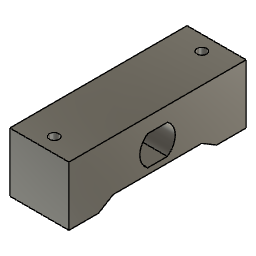
Motor mount test v1 (Autodesk Fusion 360 design; units mm, degrees)
Autodesk Fusion 360 part; units mm, degrees
sketch "Sketch1" plane through (0, 0, 0) normal (0, 0, 1) x (1, 0, 0)
  line L0 (0, 0) -> (20, 0)
  line L1 (20, 0) -> (20, 60)
  line L2 (20, 60) -> (0, 60)
  line L3 (0, 60) -> (0, 0)
  constraint horizontal L0
  constraint vertical L1
  constraint horizontal L2
  constraint vertical L3
  constraint coincident L0.start L3.end
extrude "Extrude1" add sketch "Sketch1" along normal blind 30
extrude "Extrude2" cut 1 faces at (6.6667, 40, 30) along direction (0, 0, -1) blind 10
sketch "Sketch2" plane through (20, 0, 0) normal (1, 0, 0) x (0, 1, 0)
  line L0 (60, 20) -> (0, 20)
  line L1 (0, 20) -> (0, 0)
  line L2 (0, 0) -> (60, 0)
  line L3 (60, 0) -> (60, 20)
  line L4 (36, 5) -> (24, 5)
  line L5 (24, 5) -> (24, 15)
  line L6 (24, 15) -> (36, 15)
  line L7 (36, 15) -> (36, 5)
  line L8 (36, 5) -> (24, 15) construction
  line L9 (24, 5) -> (36, 15) construction
  circle A0 centre (30, 10) radius 6
  point P0 (30, 10)
  constraint horizontal L4
  constraint perpendicular L4 L5
  constraint parallel L4 L6
  constraint parallel L5 L7
  constraint coincident L8 P0
  constraint coincident L9 P0
  constraint coincident P0 A0.centre
extrude "Extrude3" cut sketch "Sketch2" against normal blind 29 contours L4 L6 A0
sketch "Sketch3" plane through (0, 0, 0) normal (0, 0, -1) x (1, 0, 0)
  line L0 (0, 0) -> (0, -60)
  line L1 (0, -60) -> (20, -60)
  line L2 (20, -60) -> (20, 0)
  line L3 (20, 0) -> (0, 0)
  circle A0 centre (10, -5) radius 1.65
  circle A1 centre (10, -55) radius 1.65
  dimension "d7" = 3.3
  dimension "d8" = 3.3
  measures "d7" diameter of A0
  measures "d8" diameter of A1
extrude "Extrude4" cut sketch "Sketch3" against normal blind 45 contours A0 | A1
sketch "Sketch4" plane through (20, 0, 0) normal (1, 0, 0) x (0, 1, 0)
  line L0 (33.3166, 5) -> (26.6834, 5)
  arc A0 (26.6834, 15) -> (26.6834, 5) centre (30, 10) ccw
  line L1 (26.6834, 15) -> (33.3166, 15)
  arc A1 (33.3166, 5) -> (33.3166, 15) centre (30, 10) ccw
  line L2 (60, 20) -> (0, 20)
  line L3 (0, 20) -> (0, 0)
  line L4 (0, 0) -> (60, 0)
  line L5 (60, 0) -> (60, 20)
  line L6 (10, 0) -> (15, 3)
  line L7 (15, 3) -> (45, 3)
  line L8 (45, 3) -> (50, 0)
  constraint coincident L4 L6.start
  constraint parallel L4 L7
  constraint coincident L4 L8.end
extrude "Extrude5" cut sketch "Sketch4" against normal blind 43 contours L4 L6 L7 L8
